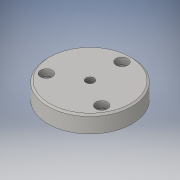
# Autodesk Inventor part: M-060-Adapter
Saved by Autodesk Inventor 2016 (Build 200138000, 138)
## iProperties
Created: 2018-11-21
Part Number: M-060-Adapter
Material: Generic
Document SubType Name: Modeling
Designer: voigt
Density: 1 g/cm^3
Appearance: Default
Author: voigt
Autodesk Inventor part; units mm, degrees
ref_plane "YZ Plane" through (0, 0, 0) normal (1, 0, 0) x (0, 1, 0)
ref_plane "XZ Plane" through (0, 0, 0) normal (0, 1, 0) x (-1, 0, 0)
ref_plane "XY Plane" through (0, 0, 0) normal (0, 0, 1) x (1, 0, 0)
sketch "Sketch1" plane through (0, 0, 0) normal (0, 0, 1) x (1, 0, 0)
  line L0 (0, 35) -> (0, -35) construction
  line L1 (-35, 0) -> (35, 0) construction
  circle A0 centre (0, 0) radius 25
  dimension "d0" = 50
  constraints: 1 centre point, 1 coincident
  measures "d0" diameter of A0
extrude "Extrusion1" add sketch "Sketch1" along normal blind 10
sketch "Sketch2" plane through (0, 0, 10) normal (0, 0, 1) x (1, 0, 0)
  point P0 (0, 0)
  point P1 (0, 0)
  constraints: 1 coincident
hole "Hole1" at (0, 0, 10) direction (0, 0, -1) diameter 4.917 end through all thread size "M6x1" class "6H" standard "ISO Metric profile"
sketch "Sketch3" plane through (0, 0, 10) normal (0, 0, 1) x (1, 0, 0)
  circle A0 centre (0, 0) radius 19 construction
  line L0 (0, 35) -> (0, -35) construction
  point P0 (0, 19)
  point P1 (-16.4545, -9.5)
  point P2 (16.4545, -9.5)
  dimension "d10" = 38
  dimension "d11" = 120
  dimension "d12" = 120
  constraints: 3 point on circle, 1 centre point, 1 coincident, 1 point on line
  measures "d10" diameter of A0
hole "Hole2" at (0, 19, 10) at (-16.4545, -9.5, 10) at (16.4545, -9.5, 10) direction (0, 0, -1) diameter 4 end through all counterbore diameter 7 counterbore depth 4
chamfer "Chamfer1" distance 1 angle 45 1 edges at (-25, 0, 10)
body "Solid1"
